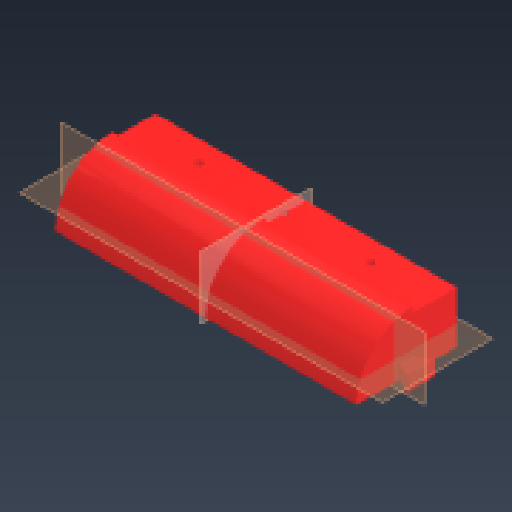
# Autodesk Inventor part: Край_новой_крышки
Saved by Autodesk Inventor 2023.2 (Build 272271030, 271C)
## iProperties
Created: 2025-10-05
Part Number: Край_новой_крышки
Material: Типовые
Document SubType Name: Modeling
Designer: Олег Коноваленко
Density: 1 g/cm^3
Appearance: Светло-красный
Author: Олег Коноваленко
Autodesk Inventor part; units mm, degrees
sketch "Эскиз1" plane through (0, 0, 0) normal (1, 0, 0) x (0, 1, 0)
  line L0 (25.8579, -14.1421) -> (-14.1421, -14.1421)
  line L1 (-14.1421, -14.1421) -> (-14.1421, 25.8579)
  arc A0 (25.8579, -14.1421) -> (-14.1421, 25.8579) centre (-14.1421, -14.1421) ccw
  line L2 (-14.1421, -14.1421) -> (14.1421, 14.1421) construction
  point P0 (0, 0)
  point P1 (0, 0)
  dimension "d0" = 40
  constraints: 6 end point, 3 point on circle, 2 line through centre, 1 centre point, 1 coincident, 1 horizontal, 1 midpoint, 1 perpendicular
  measures "d0" distance of L0.start L0.end
extrude "Выдавливание1" add sketch "Эскиз1" along normal mid plane 210
sketch "Эскиз2" plane through (105, 25.8579, -14.1421) normal (0, 0, -1) x (-1, 0, 0)
  line L0 (210, 0) -> (0, 0) projected
  line L1 (0, -40) -> (0, 0) projected
  line L2 (210, -40) -> (0, -40) projected
  line L3 (210, 0) -> (210, -40) projected
  point P0 (105, -25.8579)
extrude "Выдавливание2" add sketch "Эскиз2" along normal blind 30
sketch "Эскиз3" plane through (-105, 25.8579, -14.1421) normal (0, 1, 0) x (1, 0, 0)
  line L0 (0, 0) -> (210, 0) projected
  line L1 (210, 0) -> (210, 30) projected
  line L2 (0, 30) -> (210, 30) projected
  line L3 (0, 0) -> (0, 30) projected
  point P0 (105, -14.1421)
extrude "Выдавливание3" cut sketch "Эскиз3" against normal blind 4
sketch "Эскиз5" plane through (-105, 21.8579, -14.1421) normal (0, 1, 0) x (1, 0, 0)
  line L0 (210, -40) -> (210, 30) projected
  line L1 (210, 15) -> (0, 15) construction
  line L2 (0, -40) -> (0, 30) projected
  line L3 (0, 30) -> (210, 30) projected
  circle A0 centre (45, 15) radius 2.6
  line L4 (270, 15) -> (60, 15) construction
  circle A1 centre (105, 15) radius 2.6
  line L5 (330, 15) -> (120, 15) construction
  circle A2 centre (165, 15) radius 2.6
  dimension "d7" = 15
  dimension "d8" = 5.2
  dimension "d9" = 45
  dimension "d12" = 60
  constraints: 6 end point, 5 point on line, 3 centre point, 2 horizontal, 1 collinear, 9 other
  measures "d7" distance between parallel lines of L3 L1
  measures "d8" diameter of A0
  measures "d9" distance from line of L2 A0.centre
  measures "d12" distance of L1.start L4.start
extrude "Выдавливание4" cut sketch "Эскиз5" against normal up to next
sketch "Эскиз6" plane through (-105, -14.1421, 25.8579) normal (0, -1, 0) x (1, 0, 0)
  line L0 (-10, -25) -> (0, -30) projected
  line L1 (0, -40) -> (-10, -45) projected
  line L2 (-10, -45) -> (-10, -25) projected
  line L3 (0, 0) -> (0, -70) projected
  point P0 (105, -25.8579)
extrude "Выдавливание5" add sketch "Эскиз6" against normal blind 10
mirror "Зеркальное отражение1" about plane through (0, 0, 0) normal (1, 0, 0) of "Выдавливание5"
